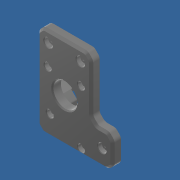
# Autodesk Inventor part: Print_Parts_D
Saved by Autodesk Inventor 2020 (Build 240168000, 168)
## iProperties
Created: 2020-09-26
Part Number: Print_Parts_D
Material: PC/ABS プラスチック
Document SubType Name: Modeling
Designer: kenta iguchi
Density: 0.357273 g/cm^3
Appearance: 滑らか - 黒
Author: kenta iguchi
Autodesk Inventor part; units mm, degrees
ref_plane "YZ Plane" through (0, 0, 0) normal (1, 0, 0) x (0, 1, 0)
ref_plane "XZ Plane" through (0, 0, 0) normal (0, 1, 0) x (-1, 0, 0)
ref_plane "XY Plane" through (0, 0, 0) normal (0, 0, 1) x (1, 0, 0)
sketch "スケッチ1" plane through (0, 0, 0) normal (0, 0, 1) x (1, 0, 0)
  line L0 (0, 0) -> (-50, 0)
  line L1 (-50, 0) -> (-50, -85)
  line L2 (-50, -85) -> (0, -85)
  line L3 (0, -85) -> (0, 0)
  dimension "d0" = 50
  dimension "d1" = 85
  constraints: 8 end point, 2 parallel, 1 horizontal, 1 perpendicular
  measures "d0" distance of L2.end L1.end
  measures "d1" distance of L1.end L0.end
extrude "押し出し1" add sketch "スケッチ1" along normal blind 8
sketch "スケッチ2" plane through (0, 0, 8) normal (0, 0, 1) x (1, 0, 0)
  line L0 (0, -85) -> (0, 0) projected
  line L1 (0, 0) -> (-50, 0) projected
  circle A0 centre (-25, -45) radius 11.15
  dimension "d4" = 45
  dimension "d5" = 25
  dimension "d6" = 22.3
  constraints: 1 centre point
  measures "d4" distance from line of A0.centre L1
  measures "d5" distance from line of L0 A0.centre
  measures "d6" diameter of A0
extrude "押し出し2" cut sketch "スケッチ2" against normal blind 10
sketch "スケッチ3" plane through (0, 0, 8) normal (0, 0, 1) x (1, 0, 0)
  circle A0 centre (-25, -45) radius 11.15 projected
  line L0 (-40.5, -60.5) -> (-9.5, -60.5)
  line L1 (-9.5, -60.5) -> (-9.5, -29.5)
  line L2 (-9.5, -29.5) -> (-40.5, -29.5)
  line L3 (-40.5, -29.5) -> (-40.5, -60.5)
  line L4 (-40.5, -60.5) -> (-9.5, -29.5) construction
  line L5 (-9.5, -60.5) -> (-40.5, -29.5) construction
  dimension "d9" = 31
  dimension "d10" = 31
  constraints: 12 end point, 2 midpoint, 2 parallel, 1 horizontal, 1 perpendicular
  measures "d9" distance of L2.end L1.end
  measures "d10" distance of L1.end L0.end
hole "穴1" at (-40.5, -29.5, 8) at (-9.5, -29.5, 8) direction (0, 0, -1) diameter 3.3 depth 58 counterbore diameter 6.5 counterbore depth 4
sketch "スケッチ4" plane through (0, 0, 0) normal (0, 0, -1) x (-1, 0, 0)
  line L0 (0, -85) -> (0, 0) projected
  line L1 (50, -85) -> (0, -85) projected
  point P0 (9.5, -80)
  point P1 (38.5, -66.5)
  dimension "d18" = 38.5
  dimension "d19" = 9.5
  dimension "d20" = 5
  dimension "d34" = 13.5
  measures "d18" distance from line of point (38.5, -66.5) L0
  measures "d19" distance from line of L0 point (9.5, -80)
  measures "d20" distance from line of point (9.5, -80) L1
  measures "d34" vertical distance of point (9.5, -80) point (38.5, -66.5)
hole "穴2" at (-9.5, -80, 0) at (-38.5, -66.5, 0) direction (0, 0, 1) diameter 3.3 depth 58
sketch "スケッチ8" plane through (0, 0, 0) normal (0, 0, -1) x (-1, 0, 0)
  circle A0 centre (38.5, -66.5) radius 1.65 projected
  line L0 (50, 0) -> (50, -85) projected
  line L1 (50, -85) -> (0, -85) projected
  line L2 (50, 0) -> (50, -85) projected
  line L3 (50, -54) -> (30.5, -54)
  line L4 (30.5, -54) -> (30.5, -70.5)
  line L5 (30.5, -70.5) -> (50, -70.5)
  line L6 (50, -70.5) -> (50, -54)
  circle A1 centre (38.5, -66.5) radius 8
  circle A2 centre (38.5, -66.5) radius 6
  circle A3 centre (38.5, -66.5) radius 4
  circle A4 centre (9.5, -80) radius 1.65 projected
  circle A5 centre (38.5, -66.5) radius 1.65 projected
  circle A6 centre (40.5, -29.5) radius 1.65 projected
  circle A7 centre (9.5, -29.5) radius 1.65 projected
  circle A8 centre (25, -45) radius 11.15 projected
  line L7 (50, 0) -> (50, -85) projected
  line L8 (0, 0) -> (50, 0) projected
  line L9 (0, -85) -> (0, 0) projected
  line L10 (50, -85) -> (0, -85) projected
  point P0 (31.582, -54)
  point P1 (30.5, -54.6991)
  dimension "d35" = 31
  dimension "d36" = 16
  dimension "d37" = 12
  dimension "d38" = 2
  constraints: 8 end point, 3 centre point, 2 coincident, 2 parallel, 2 tangent, 1 horizontal, 1 perpendicular, 1 point on line
  measures "d35" distance between parallel lines of L3 L1
  measures "d36" diameter of A1
  measures "d37" diameter of A2
  measures "d38" radial gap between concentric circles of A2 A3
extrude "押し出し5" add sketch "スケッチ8" along normal blind 10 contours L0 L5 A1 L4 A8 L3 | L5 A2 A1 | A3 | L5 A2 | L5 L4 A1 picked at (45.7558, -65.8618) picked at (43.741, -67.2784)
sketch "スケッチ9" plane through (0, 0, -10) normal (0, 0, -1) x (-1, 0, 0)
  line L0 (50, -54) -> (31.582, -54) projected
  circle A0 centre (38.5, -66.5) radius 1.65 projected
  circle A1 centre (38.5, -66.5) radius 10
  line L1 (50, -70.5) -> (36.15, -70.5)
  line L2 (36.15, -70.5) -> (36.15, -54)
  line L3 (36.15, -54) -> (50, -54)
  line L4 (50, -54) -> (50, -70.5)
  line L5 (30.5, -54.6991) -> (30.5, -70.5) projected
  line L6 (38.5, -56.5) -> (21.3308, -56.5)
  point P0 (30.5, -54)
  point P1 (0, 0)
  point P2 (36.15, -56.78)
  point P3 (47.6652, -70.5)
  point P4 (36.15, -56.5)
  dimension "d41" = 20
  dimension "d42" = 13.85
  constraints: 10 end point, 2 parallel, 2 perpendicular, 1 coincident, 1 horizontal, 1 point on line, 1 vertical alignment, 3 other
  measures "d42" distance of L2.end L3.end
extrude "押し出し6" add sketch "スケッチ9" along normal blind 10 contours L4 L1 A1 L6 L2 L0
sketch "スケッチ10" plane through (0, 0, 8) normal (0, 0, 1) x (1, 0, 0)
  line L0 (0, -85) -> (0, 0) projected
  line L1 (0, -85) -> (20, -85)
  line L2 (20, -85) -> (20, -55)
  line L3 (20, -55) -> (0, -55)
  line L4 (0, -55) -> (0, -85)
  dimension "d48" = 20
  dimension "d49" = 30
  constraints: 8 end point, 2 parallel, 1 horizontal, 1 perpendicular
  measures "d48" distance of L3.end L2.end
  measures "d49" distance of L2.end L1.end
extrude "押し出し7" add sketch "スケッチ10" against normal up to surface (8 mm away)
chamfer "面取り2" distance 5 angle 45 6 edges at (-50, -85, 4) (20, -85, 4) (20, -55, 4) (0, -55, 4) (0, 0, 4) (-50, 0, 4)
fillet "フィレット1" radius 5 12 edges at (-50, -80, 4) (-45, -85, 4) (15, -85, 4) (20, -80, 4) (20, -60, 4) (15, -55, 4) (5, -55, 4) (0, -50, 4) (0, -5, 4) (-5, 0, 4) (-45, 0, 4) (-50, -5, 4)
sketch "スケッチ11" plane through (0, 0, -10) normal (0, 0, -1) x (-1, 0, 0)
  line L0 (36.15, -56.5) -> (36.15, -54) projected
  line L1 (36.15, -54) -> (31.582, -54) projected
  arc A0 (30.5, -54.6991) -> (31.582, -54) centre (25, -45) ccw projected
  line L2 (30.5, -54.6991) -> (30.5, -70.5) projected
  line L3 (36.15, -56.5) -> (28.5102, -56.5)
  line L4 (28.5102, -56.5) -> (28.5102, -54)
  line L5 (28.5102, -54) -> (36.15, -54)
  line L6 (36.15, -54) -> (36.15, -56.5)
  point P0 (0, 0)
  point P1 (30.5, -56.5)
  constraints: 8 end point, 2 parallel, 1 horizontal, 1 horizontal alignment, 1 perpendicular
extrude "押し出し8" cut sketch "スケッチ11" against normal up to surface (10 mm away) contours L3 L2 A0 L1 L0
sketch "スケッチ12" plane through (0, 0, -10) normal (0, 0, -1) x (-1, 0, 0)
  circle A0 centre (38.5, -66.5) radius 1.65 projected
  circle A1 centre (38.5, -66.5) radius 1.65 projected
  circle A2 centre (38.5, -66.5) radius 3
  point P0 (0, 0)
  dimension "d64" = 6
  constraints: 1 centre point, 1 coincident
  measures "d64" diameter of A2
extrude "押し出し9" add sketch "スケッチ12" along normal blind 0.5
sketch "スケッチ13" plane through (0, 0, 0) normal (0, 0, -1) x (-1, 0, 0)
  circle A0 centre (9.5, -80) radius 1.65 projected
  circle A1 centre (9.5, -80) radius 3
  point P0 (0, 0)
  dimension "d70" = 6
  constraints: 1 centre point, 1 coincident
  measures "d70" diameter of A1
extrude "押し出し10" add sketch "スケッチ13" along normal blind 1
chamfer "面取り6" distance 1 angle 45 1 edges at (-6.5, -80, 0)
fillet "フィレット2" radius 1.5 1 edges at (-50, -70.5, -10)
sketch "スケッチ14" plane through (0, 0, 8) normal (0, 0, 1) x (1, 0, 0)
  circle A0 centre (-9.5, -80) radius 1.65 projected
  circle A1 centre (-38.5, -66.5) radius 1.65 projected
  point P0 (0, 0)
hole "穴3" at (-9.5, -80, 8) at (-38.5, -66.5, 8) direction (0, 0, -1) diameter 6.5 depth 4
chamfer "面取り7" distance 2 angle 45 24 edges at (-44.8423, -84.6194, 8) (-47.5, -82.5, 8) (-49.6194, -79.8423, 8) (-50, -42.5, 8) (-49.6194, -5.1577, 8) (-47.5, -2.5, 8) (-44.8423, -0.3806, 8) (-25, 0, 8) (-5.1577, -0.3806, 8) (-2.5, -2.5, 8) (-0.3806, -5.1577, 8) (0, -27.5, 8) (0.3806, -49.8423, 8) (2.5, -52.5, 8) (5.1577, -54.6194, 8) (10, -55, 8) (14.8423, -55.3806, 8) (17.5, -57.5, 8) (19.6194, -60.1577, 8) (20, -70, 8) (19.6194, -79.8423, 8) (17.5, -82.5, 8) (14.8423, -84.6194, 8) (-15, -85, 8)
sketch "スケッチ15" plane through (0, 0, 8) normal (0, 0, 1) x (1, 0, 0)
  line L0 (-7.0711, 0) -> (-42.9289, 0) projected
  arc A0 (-45.0503, -82.1213) -> (-42.9289, -83) centre (-42.9289, -80) ccw projected
  line L1 (-45.0503, -82.1213) -> (-47.1213, -80.0503) projected
  arc A1 (-48, -77.9289) -> (-47.1213, -80.0503) centre (-45, -77.9289) ccw projected
  line L2 (-48, -77.9289) -> (-48, -7.0711) projected
  arc A2 (-47.1213, -4.9497) -> (-48, -7.0711) centre (-45, -7.0711) ccw projected
  line L3 (-47.1213, -4.9497) -> (-45.0503, -2.8787) projected
  arc A3 (-42.9289, -2) -> (-45.0503, -2.8787) centre (-42.9289, -5) ccw projected
  line L4 (-42.9289, -2) -> (-7.0711, -2) projected
  arc A4 (-4.9497, -2.8787) -> (-7.0711, -2) centre (-7.0711, -5) ccw projected
  line L5 (-4.9497, -2.8787) -> (-2.8787, -4.9497) projected
  arc A5 (-2, -7.0711) -> (-2.8787, -4.9497) centre (-5, -7.0711) ccw projected
  line L6 (-2, -7.0711) -> (-2, -47.9289) projected
  arc A6 (-2, -47.9289) -> (0.0503, -52.8787) centre (5, -47.9289) ccw projected
  line L7 (0.0503, -52.8787) -> (2.1213, -54.9497) projected
  arc A7 (2.1213, -54.9497) -> (7.0711, -57) centre (7.0711, -50) ccw projected
  line L8 (7.0711, -57) -> (12.9289, -57) projected
  arc A8 (15.0503, -57.8787) -> (12.9289, -57) centre (12.9289, -60) ccw projected
  line L9 (15.0503, -57.8787) -> (17.1213, -59.9497) projected
  arc A9 (18, -62.0711) -> (17.1213, -59.9497) centre (15, -62.0711) ccw projected
  line L10 (18, -62.0711) -> (18, -77.9289) projected
  arc A10 (17.1213, -80.0503) -> (18, -77.9289) centre (15, -77.9289) ccw projected
  line L11 (17.1213, -80.0503) -> (15.0503, -82.1213) projected
  arc A11 (12.9289, -83) -> (15.0503, -82.1213) centre (12.9289, -80) ccw projected
  line L12 (12.9289, -83) -> (-8.25, -83) projected
  line L13 (-10.75, -83) -> (-42.9289, -83) projected
  circle A12 centre (-38.5, -66.5) radius 3.25 projected
  circle A13 centre (-40.5, -29.5) radius 3.25 projected
  circle A14 centre (-9.5, -29.5) radius 3.25 projected
  circle A15 centre (-25, -45) radius 11.15 projected
  line L14 (0, -47.9289) -> (0, -7.0711) projected
  line L15 (-50, -7.0711) -> (-50, -77.9289) projected
  line L16 (20, -77.9289) -> (20, -62.0711) projected
  line L17 (-42.9289, -85) -> (12.9289, -85) projected
  arc A16 (-8.25, -83) -> (-10.75, -83) centre (-9.5, -80) ccw projected
  point P0 (0, 0)
  point P1 (10, -70)
  point P2 (-10, -10)
  point P3 (-40, -10)
  dimension "d87" = 10
  dimension "d88" = 10
  dimension "d89" = 10
  dimension "d90" = 10
  dimension "d91" = 15
  constraints: 1 horizontal alignment
  measures "d87" distance from line of point (-10, -10) L14
  measures "d88" distance from line of point (-40, -10) L0
  measures "d89" distance from line of point (-40, -10) L15
  measures "d90" distance from line of point (10, -70) L16
  measures "d91" distance from line of point (10, -70) L17
hole "穴4" at (10, -70, 8) at (-10, -10, 8) at (-40, -10, 8) direction (0, 0, -1) diameter 4.3 end through all counterbore diameter 8 counterbore depth 4
sketch "スケッチ16" plane through (-40, -10, 4) normal (0, 0, 1) x (1, 0, 0)
  circle A0 centre (30, 0) radius 4 projected
  circle A1 centre (30, 0) radius 2.15 projected
  circle A2 centre (50, -60) radius 4 projected
  circle A3 centre (50, -60) radius 2.15 projected
  circle A4 centre (0, 0) radius 4 projected
  circle A5 centre (0, 0) radius 2.15 projected
  circle A6 centre (15, -35) radius 11.15 projected
  arc A7 (36.4645, 8.5355) -> (32.9289, 10) centre (32.9289, 5) ccw projected
  line L0 (36.4645, 8.5355) -> (38.5355, 6.4645) projected
  arc A8 (40, 2.9289) -> (38.5355, 6.4645) centre (35, 2.9289) ccw projected
  line L1 (40, 2.9289) -> (40, -37.9289) projected
  arc A9 (40, -37.9289) -> (41.4645, -41.4645) centre (45, -37.9289) ccw projected
  line L2 (41.4645, -41.4645) -> (43.5355, -43.5355) projected
  arc A10 (43.5355, -43.5355) -> (47.0711, -45) centre (47.0711, -40) ccw projected
  line L3 (47.0711, -45) -> (52.9289, -45) projected
  arc A11 (56.4645, -46.4645) -> (52.9289, -45) centre (52.9289, -50) ccw projected
  line L4 (56.4645, -46.4645) -> (58.5355, -48.5355) projected
  arc A12 (60, -52.0711) -> (58.5355, -48.5355) centre (55, -52.0711) ccw projected
  line L5 (60, -52.0711) -> (60, -67.9289) projected
  arc A13 (58.5355, -71.4645) -> (60, -67.9289) centre (55, -67.9289) ccw projected
  line L6 (58.5355, -71.4645) -> (56.4645, -73.5355) projected
  arc A14 (52.9289, -75) -> (56.4645, -73.5355) centre (52.9289, -70) ccw projected
  line L7 (52.9289, -75) -> (-2.9289, -75) projected
  arc A15 (-6.4645, -73.5355) -> (-2.9289, -75) centre (-2.9289, -70) ccw projected
  line L8 (-6.4645, -73.5355) -> (-8.5355, -71.4645) projected
  arc A16 (-10, -67.9289) -> (-8.5355, -71.4645) centre (-5, -67.9289) ccw projected
  line L9 (-10, -67.9289) -> (-10, 2.9289) projected
  arc A17 (-8.5355, 6.4645) -> (-10, 2.9289) centre (-5, 2.9289) ccw projected
  line L10 (-8.5355, 6.4645) -> (-6.4645, 8.5355) projected
  arc A18 (-2.9289, 10) -> (-6.4645, 8.5355) centre (-2.9289, 5) ccw projected
  line L11 (-2.9289, 10) -> (32.9289, 10) projected
  line L12 (-2.15, -2.15) -> (2.15, -2.15)
  line L13 (2.15, -2.15) -> (2.15, 2.15)
  line L14 (2.15, 2.15) -> (-2.15, 2.15)
  line L15 (-2.15, 2.15) -> (-2.15, -2.15)
  circle A19 centre (0, 0) radius 2.15 projected
  line L16 (-2.15, -2.15) -> (2.15, 2.15) construction
  line L17 (2.15, -2.15) -> (-2.15, 2.15) construction
  line L18 (-2.15, -21.15) -> (1.15, -21.15)
  line L19 (1.15, -21.15) -> (1.15, -17.85)
  line L20 (1.15, -17.85) -> (-2.15, -17.85)
  line L21 (-2.15, -17.85) -> (-2.15, -21.15)
  line L22 (-2.15, -21.15) -> (1.15, -17.85) construction
  line L23 (1.15, -21.15) -> (-2.15, -17.85) construction
  line L24 (-0.15, -58.15) -> (3.15, -58.15)
  line L25 (3.15, -58.15) -> (3.15, -54.85)
  line L26 (3.15, -54.85) -> (-0.15, -54.85)
  line L27 (-0.15, -54.85) -> (-0.15, -58.15)
  circle A20 centre (1.5, -56.5) radius 1.65 projected
  line L28 (-0.15, -58.15) -> (3.15, -54.85) construction
  line L29 (3.15, -58.15) -> (-0.15, -54.85) construction
  line L30 (28.85, -71.65) -> (32.15, -71.65)
  line L31 (32.15, -71.65) -> (32.15, -68.35)
  line L32 (32.15, -68.35) -> (28.85, -68.35)
  line L33 (28.85, -68.35) -> (28.85, -71.65)
  circle A21 centre (30.5, -70) radius 1.65 projected
  line L34 (28.85, -71.65) -> (32.15, -68.35) construction
  line L35 (32.15, -71.65) -> (28.85, -68.35) construction
  line L36 (47.85, -62.15) -> (52.15, -62.15)
  line L37 (52.15, -62.15) -> (52.15, -57.85)
  line L38 (52.15, -57.85) -> (47.85, -57.85)
  line L39 (47.85, -57.85) -> (47.85, -62.15)
  circle A22 centre (50, -60) radius 4 projected
  line L40 (47.85, -62.15) -> (52.15, -57.85) construction
  line L41 (52.15, -62.15) -> (47.85, -57.85) construction
  line L42 (28.85, -21.15) -> (32.15, -21.15)
  line L43 (32.15, -21.15) -> (32.15, -17.85)
  line L44 (32.15, -17.85) -> (28.85, -17.85)
  line L45 (28.85, -17.85) -> (28.85, -21.15)
  line L46 (28.85, -21.15) -> (32.15, -17.85) construction
  line L47 (32.15, -21.15) -> (28.85, -17.85) construction
  line L48 (27.85, -2.15) -> (32.15, -2.15)
  line L49 (32.15, -2.15) -> (32.15, 2.15)
  line L50 (32.15, 2.15) -> (27.85, 2.15)
  line L51 (27.85, 2.15) -> (27.85, -2.15)
  line L52 (27.85, -2.15) -> (32.15, 2.15) construction
  line L53 (32.15, -2.15) -> (27.85, 2.15) construction
  circle A23 centre (30.5, -70) radius 3.25 projected
  circle A24 centre (1.5, -56.5) radius 3.25 projected
  circle A25 centre (30.5, -70) radius 1.65 projected
  circle A26 centre (1.5, -56.5) radius 1.65 projected
  circle A27 centre (-0.5, -19.5) radius 3.25 projected
  circle A28 centre (-0.5, -19.5) radius 1.65 projected
  circle A29 centre (30.5, -19.5) radius 3.25 projected
  circle A30 centre (30.5, -19.5) radius 1.65 projected
  point P0 (40, 10)
  constraints: 84 end point, 14 midpoint, 14 parallel, 7 horizontal, 7 perpendicular, 4 point on line
extrude "押し出し11" cut sketch "スケッチ16" against normal blind 0.6 contours A1 | L49 L48 A1 | A1 L50 L49 | A1 L51 L50 | L48 L51 A1 | A3 | L37 L36 A3 | A3 L38 L37 | A3 L39 L38 | L36 L39 A3 | A5 | L13 L12 A5 | A5 L14 L13 | A5 L15 L14 | L12 L15 A5 | L21 A28 L18 | A28 L19 L18 | A28 | L21 L20 A28 | A28 L20 L19 | L27 A20 L24 | A20 L25 L24 | A20 | L27 L26 A20 | A20 L26 L25 | L33 A21 L30 | A21 L31 L30 | A21 | L33 L32 A21 | A21 L32 L31 | L45 A30 L42 | A30 L43 L42 | A30 | L45 L44 A30 | A30 L44 L43
sketch "スケッチ17" plane through (-40.5, -29.5, 4) normal (0, 0, 1) x (1, 0, 0)
  line L0 (-1.65, 1.65) -> (1.65, 1.65) projected
  line L1 (1.65, -1.65) -> (-1.65, -1.65) projected
  circle A0 centre (0, 0) radius 3.25 projected
  line L2 (-1.65, 17.35) -> (-1.65, 21.65) projected
  line L3 (-1.65, 21.65) -> (2.65, 21.65) projected
  line L4 (2.65, 21.65) -> (2.65, 17.35) projected
  line L5 (2.65, 17.35) -> (-1.65, 17.35) projected
  circle A1 centre (0.5, 19.5) radius 4 projected
  line L6 (32.65, 21.65) -> (32.65, 17.35) projected
  line L7 (32.65, 17.35) -> (28.35, 17.35) projected
  line L8 (28.35, 17.35) -> (28.35, 21.65) projected
  line L9 (28.35, 21.65) -> (32.65, 21.65) projected
  circle A2 centre (30.5, 19.5) radius 4 projected
  circle A3 centre (31, 0) radius 3.25 projected
  line L10 (52.65, -38.35) -> (52.65, -42.65) projected
  line L11 (52.65, -42.65) -> (48.35, -42.65) projected
  line L12 (48.35, -42.65) -> (48.35, -38.35) projected
  line L13 (48.35, -38.35) -> (52.65, -38.35) projected
  circle A4 centre (50.5, -40.5) radius 4 projected
  circle A5 centre (31, -50.5) radius 3 projected
  circle A6 centre (2, -37) radius 3.25 projected
  circle A7 centre (0.5, 19.5) radius 4 projected
  line L14 (-1.65, 16.1269) -> (2.65, 16.1269)
  line L15 (2.65, 16.1269) -> (2.65, 22.8731)
  line L16 (2.65, 22.8731) -> (-1.65, 22.8731)
  line L17 (-1.65, 22.8731) -> (-1.65, 16.1269)
  line L18 (-1.65, 16.1269) -> (2.65, 22.8731) construction
  line L19 (2.65, 16.1269) -> (-1.65, 22.8731) construction
  circle A8 centre (0, 0) radius 3.25 projected
  line L20 (-1.65, -2.8) -> (1.65, -2.8)
  line L21 (1.65, -2.8) -> (1.65, 2.8)
  line L22 (1.65, 2.8) -> (-1.65, 2.8)
  line L23 (-1.65, 2.8) -> (-1.65, -2.8)
  line L24 (-1.65, -2.8) -> (1.65, 2.8) construction
  line L25 (1.65, -2.8) -> (-1.65, 2.8) construction
  circle A9 centre (2, -37) radius 3.25 projected
  line L26 (0.35, -39.8) -> (3.65, -39.8)
  line L27 (3.65, -39.8) -> (3.65, -34.2)
  line L28 (3.65, -34.2) -> (0.35, -34.2)
  line L29 (0.35, -34.2) -> (0.35, -39.8)
  line L30 (0.35, -39.8) -> (3.65, -34.2) construction
  line L31 (3.65, -39.8) -> (0.35, -34.2) construction
  line L32 (29.35, -53.3) -> (32.65, -53.3)
  line L33 (32.65, -53.3) -> (32.65, -47.7)
  line L34 (32.65, -47.7) -> (29.35, -47.7)
  line L35 (29.35, -47.7) -> (29.35, -53.3)
  line L36 (29.35, -53.3) -> (32.65, -47.7) construction
  line L37 (32.65, -53.3) -> (29.35, -47.7) construction
  circle A10 centre (50.5, -40.5) radius 4 projected
  line L38 (48.35, -43.8731) -> (52.65, -43.8731)
  line L39 (52.65, -43.8731) -> (52.65, -37.1269)
  line L40 (52.65, -37.1269) -> (48.35, -37.1269)
  line L41 (48.35, -37.1269) -> (48.35, -43.8731)
  line L42 (48.35, -43.8731) -> (52.65, -37.1269) construction
  line L43 (52.65, -43.8731) -> (48.35, -37.1269) construction
  circle A11 centre (31, -50.5) radius 3.25 projected
  arc A12 (32.25, -53.5) -> (29.75, -53.5) centre (31, -50.5) ccw projected
  circle A13 centre (31, 0) radius 3.25 projected
  line L44 (32.65, -2.8) -> (29.35, -2.8)
  line L45 (29.35, -2.8) -> (29.35, 2.8)
  line L46 (29.35, 2.8) -> (32.65, 2.8)
  line L47 (32.65, 2.8) -> (32.65, -2.8)
  line L48 (32.65, -2.8) -> (29.35, 2.8) construction
  line L49 (29.35, -2.8) -> (32.65, 2.8) construction
  circle A14 centre (30.5, 19.5) radius 4 projected
  line L50 (32.65, 16.1269) -> (28.35, 16.1269)
  line L51 (28.35, 16.1269) -> (28.35, 22.8731)
  line L52 (28.35, 22.8731) -> (32.65, 22.8731)
  line L53 (32.65, 22.8731) -> (32.65, 16.1269)
  line L54 (32.65, 16.1269) -> (28.35, 22.8731) construction
  line L55 (28.35, 16.1269) -> (32.65, 22.8731) construction
  point P0 (40.5, 29.5)
  point P1 (32.65, 2.8)
  point P2 (29.35, 2.8)
  point P3 (2.65, 22.8731)
  point P4 (2.65, 16.1269)
  point P5 (-1.65, 2.8)
  point P6 (1.65, 2.8)
  point P7 (-1.65, -2.8)
  point P8 (1.65, -2.8)
  point P9 (32.65, -53.3)
  point P10 (29.35, -53.3)
  point P11 (29.35, -47.7)
  point P12 (32.65, -47.7)
  point P13 (0.35, -35.35)
  point P14 (29.35, -48.85)
  point P15 (29.35, 1.65)
  constraints: 84 end point, 14 midpoint, 14 parallel, 7 horizontal, 7 perpendicular, 7 point on circle, 5 vertical alignment
extrude "押し出し12" cut sketch "スケッチ17" against normal blind 0.3 contours L23 L22 L21 L0 | A0 L22 | L1 L21 L20 L23 | L20 A0 | L5 L15 L14 L17 | L17 L16 L15 L3 | L14 A1 | A1 L16 | L9 L51 L52 L53 | L53 L50 L51 L7 | L52 A2 | A2 L50 | L46 A3 | L47 L44 L45 L46 | A3 L44 | L13 L41 L40 L39 | L39 L38 L41 L11 | L40 A4 | A4 L38 | L33 A5 L32 L35 L34 | A5 L34 L33 | L33 L32 A5 | L34 A5 | A5 L34 A11 | L32 A11 A5 | A5 L32 | A5 L35 L34 | L32 L35 A5 | L28 A6 | L27 L26 L29 L28 | A6 L26
chamfer "面取り8" distance 0.5 angle 45 7 edges at (-10, -6, 8) (-9.5, -26.25, 8) (-40.5, -26.25, 8) (-38.5, -63.25, 8) (-9.5, -76.75, 8) (10, -66, 8) (-40, -6, 8)
chamfer "面取り10" distance 2.5 angle 45 1 edges at (-36.15, -56.5, -5)
sketch "スケッチ19" plane through (0, 0, -10) normal (0, 0, -1) x (-1, 0, 0)
  line L0 (33.65, -56.5) -> (30.5, -56.5) projected
  line L1 (30.5, -56.5) -> (30.5, -70.5) projected
  line L2 (36.15, -54) -> (33.65, -56.5) projected
  line L3 (33.65, -56.5) -> (30.5, -59.65)
  line L4 (30.5, -70.5) -> (30.5, -56.5) projected
  point P0 (0, 0)
  constraints: 2 end point, 1 collinear, 1 point on line
extrude "押し出し14" cut sketch "スケッチ19" against normal up to surface (10 mm away)
fillet "フィレット3" radius 2 2 edges at (-30.5, -59.65, -5) (-30.5, -70.5, -5)
sketch "スケッチ20" plane through (0, 0, -20) normal (0, 0, -1) x (-1, 0, 0)
  line L0 (47.6652, -70.5) -> (48.5, -70.5) projected
  line L1 (32.5, -70.5) -> (47.6652, -70.5) projected
  arc A0 (47.6652, -70.5) -> (38.5, -56.5) centre (38.5, -66.5) ccw projected
  line L2 (47.6652, -70.5) -> (48.5, -70.5)
  line L3 (48.5, -70.5) -> (48.5, -66.5)
  line L4 (48.5, -66.5) -> (47.6652, -66.5)
  line L5 (47.6652, -66.5) -> (47.6652, -70.5)
  point P0 (0, 0)
  constraints: 8 end point, 2 parallel, 1 horizontal, 1 perpendicular, 1 point on circle
extrude "押し出し15" cut sketch "スケッチ20" against normal up to surface (10 mm away)
sketch "スケッチ21" plane through (0, 0, -10) normal (0, 0, -1) x (-1, 0, 0)
  arc A0 (48.5, -66.5) -> (38.5, -56.5) centre (38.5, -66.5) ccw projected
  line L0 (38.5, -56.5) -> (36.15, -56.5) projected
  line L1 (36.15, -54) -> (36.15, -56.5) projected
  line L2 (36.15, -54) -> (31.0858, -59.0642) projected
  arc A1 (31.0858, -59.0642) -> (30.5, -60.4784) centre (32.5, -60.4784) ccw projected
  line L3 (30.5, -60.4784) -> (30.5, -68.5) projected
  arc A2 (30.5, -68.5) -> (32.5, -70.5) centre (32.5, -68.5) ccw projected
  line L4 (32.5, -70.5) -> (48.5, -70.5) projected
  line L5 (48.5, -66.5) -> (48.5, -70.5) projected
  circle A3 centre (38.5, -66.5) radius 3 projected
  point P0 (0, 0)
  point P1 (38.5, -64.85)
extrude "押し出し16" cut sketch "スケッチ21" against normal blind 0.5
chamfer "面取り11" distance 1 angle 45 1 edges at (-35.5, -66.5, -9.5)
chamfer "面取り12" distance 1 angle 45 1 edges at (-36.15, -45, 8)
